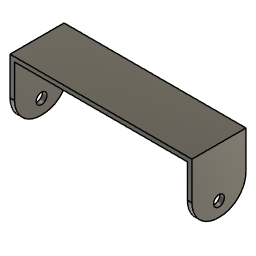
Z rotation double servo v8 (Autodesk Fusion 360 design; units mm, degrees)
Autodesk Fusion 360 part; units mm, degrees
note: some values were not read from the file. Set by a fixed rule: which sketch regions a step uses.
sketch "Sketch1" plane through (0, 0, 0) normal (0, 0, 1) x (1, 0, 0)
  line L0 (-48, 15) -> (48, 15)
  line L1 (48, 15) -> (48, -15)
  line L2 (48, -15) -> (-48, -15)
  line L3 (-48, -15) -> (-48, 15)
  line L4 (-48, 15) -> (48, -15) construction
  line L5 (48, 15) -> (-48, -15) construction
  line L6 (50.5, 15) -> (48, 15)
  line L7 (48, 15) -> (48, -15)
  line L8 (48, -15) -> (50.5, -15)
  line L9 (50.5, -15) -> (50.5, 15)
  line L10 (-50.5, -15) -> (-48, -15)
  line L11 (-48, -15) -> (-48, 15)
  line L12 (-48, 15) -> (-50.5, 15)
  line L13 (-50.5, 15) -> (-50.5, -15)
  dimension "d1" = 96
  dimension "d2" = 30
  dimension "d8" = 2.5
  dimension "d9" = 2.5
  constraint horizontal L0
  constraint perpendicular L0 L1
  constraint parallel L0 L2
  constraint parallel L1 L3
  constraint coincident L4 origin
  constraint coincident L5 origin
  constraint horizontal L6
  constraint vertical L7
  constraint horizontal L8
  constraint vertical L9
  constraint coincident L0 L6.start
  constraint horizontal L10
  constraint vertical L11
  constraint horizontal L12
  constraint vertical L13
  constraint coincident L2 L10.start
  measures "d1" distance of L1.end L2.end
  measures "d2" distance of L0.end L1.end
  measures "d8" distance of L1.end L8.end
  measures "d9" distance of L10.start L2.end
extrude "Extrude1" add sketch "Sketch1" against normal blind 23 contours L3 L10 L11 L12 L13 | L1 L6 L7 L8 L9 makes body 1 at (50.5, -5, -7.6667) makes body 2 at (-48, 5, -15.3333)
extrude "Extrude2" add sketch "Sketch1" along normal blind 2.5 bodies 1 2
sketch "Sketch2" plane through (-50.5, 0, 0) normal (-1, 0, 0) x (0, -1, 0)
  line L0 (-15, 2.5) -> (-15, -23)
  line L1 (-15, -23) -> (15, -23)
  line L2 (15, -23) -> (15, 2.5)
  line L3 (15, 2.5) -> (-15, 2.5)
  circle A0 centre (0, -15) radius 3
  dimension "d10" = 6
  measures "d10" diameter of A0
extrude "Extrude3" cut sketch "Sketch2" against normal blind 175 contours A0 bodies 1
fillet "Fillet1" radius 14.5 4 edges at (-49.25, -15, -23) (-49.25, 15, -23) (49.25, 15, -23) (49.25, -15, -23) on bodies 1
extrude "Extrude4" add 1 faces at (-16.8333, -5, 2.5) along direction (0, 0, 1) blind 10 on bodies 1 bodies 1
extrude "Extrude5" cut sketch "Sketch1" along normal blind 10 contours L0 L1 L2 L3 L7 L11 bodies 1
